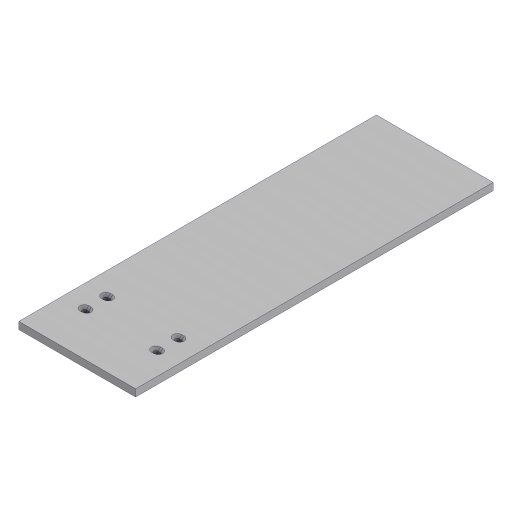
# Autodesk Inventor part: I Türe
Saved by Autodesk Inventor 2023 (Build 270158000, 158)
## iProperties
Created: 2022-09-18
Part Number: I Türe
Material: PVC, hart
Document SubType Name: Modeling
Designer: musati
Density: 1.29 g/cm^3
Appearance: Violett
Author: musati
Autodesk Inventor part; units mm, degrees
ref_plane "YZ Plane" through (0, 0, 0) normal (1, 0, 0) x (0, 1, 0)
ref_plane "XZ Plane" through (0, 0, 0) normal (0, 1, 0) x (-1, 0, 0)
ref_plane "XY Plane" through (0, 0, 0) normal (0, 0, 1) x (1, 0, 0)
sketch "Skizze1" plane through (0, 0, 0) normal (0, 0, 1) x (1, 0, 0)
  line L0 (-68.6, 0) -> (68.6, 0) projected
  line L1 (0, -4.2) -> (0, 4.2) projected
  line L2 (-49, -3) -> (49, -3)
  line L3 (49, -3) -> (49, 3)
  line L4 (49, 3) -> (-49, 3)
  line L5 (-49, 3) -> (-49, -3)
  line L6 (-49, -3) -> (49, 3) construction
  line L7 (49, -3) -> (-49, 3) construction
  point P0 (0, 0)
  dimension "d0" = 98
  dimension "d1" = 6
  constraints: 12 end point, 2 midpoint, 2 parallel, 1 horizontal, 1 perpendicular
  measures "d0" distance of L4.end L3.end
  measures "d1" distance of L3.end L2.end
extrude "Extrusion1" add sketch "Skizze1" against normal blind 300
sketch "Skizze2" plane through (-49, 3, 0) normal (0, 1, 0) x (1, 0, 0)
  line L0 (-19.6, 0) -> (117.6, 0) projected
  line L1 (49, 360) -> (49, -60) projected
  line L2 (98, 0) -> (0, 0) projected
  line L3 (98, 0) -> (98, 300) projected
  line L4 (0, 300) -> (98, 300) projected
  line L5 (0, 0) -> (0, 300) projected
  line L6 (18, 37) -> (20, 37) construction
  line L7 (18, 35.25) -> (20, 35.25)
  line L8 (20, 38.75) -> (18, 38.75)
  arc A0 (18, 38.75) -> (18, 35.25) centre (18, 37) ccw
  arc A1 (20, 35.25) -> (20, 38.75) centre (20, 37) ccw
  arc A2 (20, 53.25) -> (20, 56.75) centre (20, 55) ccw
  line L9 (18, 53.25) -> (20, 53.25)
  arc A3 (18, 56.75) -> (18, 53.25) centre (18, 55) ccw
  line L10 (20, 56.75) -> (18, 56.75)
  arc A4 (80, 35.25) -> (80, 38.75) centre (80, 37) ccw
  line L11 (78, 35.25) -> (80, 35.25)
  arc A5 (78, 38.75) -> (78, 35.25) centre (78, 37) ccw
  line L12 (80, 38.75) -> (78, 38.75)
  arc A6 (80, 53.25) -> (80, 56.75) centre (80, 55) ccw
  line L13 (78, 53.25) -> (80, 53.25)
  arc A7 (78, 56.75) -> (78, 53.25) centre (78, 55) ccw
  line L14 (80, 56.75) -> (78, 56.75)
  point P0 (49, 0)
  point P1 (19, 37)
  dimension "d4" = 2
  dimension "d5" = 3.5
  dimension "d8" = 18
  dimension "d11" = 60
  dimension "d14" = 37
  constraints: 20 end point, 16 point on circle, 8 centre point, 4 tangent, 2 horizontal, 1 midpoint, 1 parallel, 1 vertical, 31 other
  measures "d4" distance of L6.start L6.end
  measures "d5" diameter of A1
  measures "d8" distance of L6.end A2.centre
  measures "d11" distance of L6.end A4.centre
  measures "d14" distance from line of point (19, 37) L0
extrude "Extrusion2" cut sketch "Skizze2" against normal blind 300 contours A0 L8 A1 L7 | L9 A3 L10 A2 | L11 A5 L12 A4 | L13 A7 L14 A6
chamfer "Fase1" distance 2 angle 45 16 edges at (-27.25, 3, -37) (-30, 3, -35.25) (-32.75, 3, -37) (-30, 3, -38.75) (-27.25, 3, -55) (-30, 3, -53.25) (-32.75, 3, -55) (-30, 3, -56.75) (30, 3, -35.25) (27.25, 3, -37) (30, 3, -38.75) (32.75, 3, -37) (32.75, 3, -55) (30, 3, -53.25) (27.25, 3, -55) (30, 3, -56.75)
